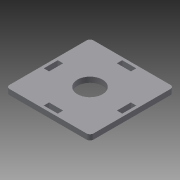
# Autodesk Inventor part: top
Saved by Autodesk Inventor 2015 SP1 (Build 190203100, 203)
## iProperties
Created: 2016-04-13
Part Number: top
Material: Generic
Document SubType Name: Modeling
Designer: tuttlem
Density: 1 g/cm^3
Appearance: Default
Author: tuttlem
Autodesk Inventor part; units mm, degrees
ref_plane "YZ Plane" through (0, 0, 0) normal (1, 0, 0) x (0, 1, 0)
ref_plane "XZ Plane" through (0, 0, 0) normal (0, 1, 0) x (-1, 0, 0)
ref_plane "XY Plane" through (0, 0, 0) normal (0, 0, 1) x (1, 0, 0)
sketch "Sketch1" plane through (0, 0, 0) normal (0, 1, 0) x (-1, 0, 0)
  line L0 (0, 0) -> (-76.2, 0)
  line L1 (-76.2, 0) -> (-76.2, -76.2)
  line L2 (-76.2, -76.2) -> (0, -76.2)
  line L3 (0, -76.2) -> (0, 0)
  line L4 (-44.45, -73.66) -> (-31.75, -73.66)
  line L5 (-31.75, -73.66) -> (-31.75, -68.834)
  line L6 (-31.75, -68.834) -> (-44.45, -68.834)
  line L7 (-44.45, -68.834) -> (-44.45, -73.66)
  line L8 (-68.834, -31.75) -> (-68.834, -44.45)
  line L9 (-68.834, -44.45) -> (-73.66, -44.45)
  line L10 (-73.66, -31.75) -> (-68.834, -31.75)
  line L11 (-73.66, -44.45) -> (-73.66, -31.75)
  line L12 (-7.366, -44.45) -> (-2.54, -44.45)
  line L13 (-7.366, -31.75) -> (-7.366, -44.45)
  line L14 (-2.54, -44.45) -> (-2.54, -31.75)
  line L15 (-2.54, -31.75) -> (-7.366, -31.75)
  line L16 (-44.45, -2.54) -> (-31.75, -2.54)
  line L17 (-31.75, -2.54) -> (-31.75, -7.366)
  line L18 (-31.75, -7.366) -> (-44.45, -7.366)
  line L19 (-44.45, -7.366) -> (-44.45, -2.54)
  circle A0 centre (-38.1, -38.1) radius 11.43
  dimension "d0" = 76.2
  dimension "d1" = 76.2
  dimension "d6" = 31.75
  dimension "d7" = 2.54
  dimension "d8" = 4.826
  dimension "d9" = 12.7
  dimension "d15" = 31.75
  dimension "d16" = 12.7
  dimension "d17" = 4.826
  dimension "d18" = 22.86
  constraints: 40 end point, 2 parallel, 1 centre point, 1 horizontal, 1 perpendicular
  measures "d0" distance of L2.end L1.end
  measures "d1" distance of L1.end L0.end
  measures "d6" distance from line of L10 L0.end
  measures "d7" distance between parallel lines of L11 L1
  measures "d8" distance of L9.start L9.end
  measures "d9" distance of L8.start L9.start
  measures "d15" distance between parallel lines of L3 L5
  measures "d16" distance of L5.end L6.end
  measures "d17" distance of L6.end L4.start
  measures "d18" diameter of A0
extrude "Extrusion3" add sketch "Sketch1" along normal blind 4.826
fillet "Fillet1" radius 3.175 4 edges at (76.2, 2.413, 0) (0, 2.413, 0) (76.2, 2.413, -76.2) (0, 2.413, -76.2)
body "Solid2"
